Autodesk Inventor part; units mm, degrees
(part 2 of 5)
  spline S5 degree 5 poles (3.499, 4.4219) (3.499, 4.422) (3.4991, 4.4221) (3.4992, 4.4222) (3.4994, 4.4225) (3.4998, 4.423) (3.5001, 4.4234) (3.5005, 4.424) (3.501, 4.4246) (3.5015, 4.4253) (3.502, 4.426) (3.5026, 4.4268) (3.5032, 4.4277) (3.5039, 4.4286) (3.5046, 4.4296) (3.5053, 4.4307) (3.5061, 4.4318) (3.5069, 4.433) (3.5077, 4.4342) (3.5086, 4.4355) (3.5095, 4.4369) (3.5104, 4.4383) (3.5114, 4.4398) (3.5124, 4.4413) (3.5135, 4.4429) (3.5145, 4.4446) (3.5156, 4.4463) (3.5168, 4.4481) (3.5179, 4.4499) (3.5191, 4.4518) (3.5203, 4.4538) (3.5215, 4.4558) (3.5231, 4.4583) (3.5246, 4.4609) (3.5262, 4.4635) (3.5281, 4.4667) (3.53, 4.4701) (3.5317, 4.473) (3.5337, 4.4765) (3.5358, 4.4802) (3.5376, 4.4834) (3.5394, 4.4867) (3.5416, 4.4906) (3.5444, 4.4958) (3.5473, 4.5012) (3.5502, 4.5068) (3.5532, 4.5125) (3.5562, 4.5185) (3.5586, 4.5232) (3.561, 4.528) (3.5635, 4.533) (3.5663, 4.5387) (3.5687, 4.5439) (3.5709, 4.5484) (3.5734, 4.5538) (3.5759, 4.5592) (3.5781, 4.564) (3.5807, 4.5696) (3.5832, 4.5753) (3.5855, 4.5803) (3.5881, 4.5862) (3.5907, 4.5923) (3.5929, 4.5975) (3.5955, 4.6037) (3.5982, 4.61) (3.6004, 4.6155) (3.6031, 4.6219) (3.6057, 4.6285) (3.608, 4.6342) (3.6107, 4.641) (3.6133, 4.6478) (3.6156, 4.6537) (3.6183, 4.6607) (3.6209, 4.6679) (3.6232, 4.674) (3.6259, 4.6813) (3.6285, 4.6887) (3.6308, 4.6951) (3.6335, 4.7026) (3.6361, 4.7102) (3.6384, 4.7168) (3.641, 4.7246) (3.6437, 4.7325) (3.6459, 4.7393) (3.6485, 4.7474) (3.6511, 4.7555) (3.6533, 4.7626) (3.6559, 4.7708) (3.6585, 4.7792) (3.6607, 4.7865) (3.6632, 4.795) (3.6658, 4.8036) (3.6679, 4.8111) (3.6705, 4.8199) (3.6729, 4.8288) (3.6751, 4.8364) (3.6775, 4.8454) (3.68, 4.8545) (3.6821, 4.8624) (3.6845, 4.8717) (3.6869, 4.881) (3.6889, 4.8891) (3.6912, 4.8985) (3.6936, 4.9081) (3.6956, 4.9164) (3.6978, 4.9261) (3.7001, 4.9359) (3.702, 4.9443) (3.7043, 4.9543) (3.7065, 4.9643) (3.7083, 4.9729) (3.7105, 4.9831) (3.7126, 4.9933) (3.7144, 5.0021) (3.7165, 5.0125) (3.7185, 5.023) (3.7202, 5.032) (3.7222, 5.0425) (3.7242, 5.0532) (3.7258, 5.0624) (3.7277, 5.0732) (3.7296, 5.0841) (3.7312, 5.0934) (3.733, 5.1044) (3.7348, 5.1155) (3.7363, 5.1251) (3.738, 5.1363) (3.7397, 5.1475) (3.7411, 5.1572) (3.7427, 5.1686) (3.7443, 5.1801) (3.7456, 5.19) (3.7472, 5.2016) (3.7486, 5.2133) (3.7499, 5.2233) (3.7513, 5.2351) (3.7527, 5.247) (3.7538, 5.2572) (3.7551, 5.2692) (3.7564, 5.2812) (3.7574, 5.2916) (3.7586, 5.3037) (3.7598, 5.316) (3.7607, 5.3265) (3.7618, 5.3388) (3.7628, 5.3513) (3.7637, 5.3619) (3.7648, 5.3763) (3.7658, 5.3907) (3.7667, 5.4033) (3.7675, 5.4161) (3.7682, 5.4289) (3.7691, 5.4435) (3.7698, 5.4583) (3.7705, 5.4731) (3.7712, 5.4881) (3.7718, 5.505) (3.7722, 5.5163) (3.7726, 5.5276) (3.773, 5.5428) (3.7734, 5.5581) (3.7736, 5.5715) (3.7738, 5.585) (3.774, 5.5985) (3.7741, 5.6082) (3.7741, 5.6179) (3.7742, 5.6277) (3.7742, 5.6375) (3.7742, 5.6473) (3.7742, 5.6571) (3.7741, 5.667) (3.774, 5.6769) (3.7739, 5.6868) (3.7738, 5.6967) (3.7736, 5.7067) (3.7734, 5.7167) (3.7732, 5.7267) (3.7729, 5.7368) (3.7727, 5.7468) (3.7724, 5.757) (3.772, 5.7671) (3.7717, 5.7772) (3.7713, 5.7874) (3.7709, 5.7976) (3.7705, 5.8079) (3.77, 5.8181) (3.7695, 5.8284) (3.769, 5.8387) (3.7685, 5.849) (3.7677, 5.8635) (3.7669, 5.876) (3.7663, 5.8864) (3.7657, 5.8948) (3.7653, 5.901) knots 0 0 0 0 0 0 0.004167 0.008333 0.0125 0.016667 0.020833 0.025 0.029167 0.033333 0.0375 0.041667 0.045833 0.05 0.054167 0.058333 0.0625 0.066667 0.070833 0.075 0.079167 0.083333 0.0875 0.091667 0.095833 0.1 0.104167 0.108333 0.1125 0.116667 0.120833 0.125 0.129167 0.1375 0.141667 0.145833 0.154167 0.158333 0.1625 0.170833 0.175 0.179167 0.183333 0.191667 0.208333 0.2125 0.216667 0.220833 0.229167 0.2375 0.241667 0.245833 0.254167 0.258333 0.2625 0.270833 0.275 0.279167 0.2875 0.291667 0.295833 0.304167 0.308333 0.3125 0.320833 0.325 0.329167 0.3375 0.341667 0.345833 0.354167 0.358333 0.3625 0.370833 0.375 0.379167 0.3875 0.391667 0.395833 0.404167 0.408333 0.4125 0.420833 0.425 0.429167 0.4375 0.441667 0.445833 0.454167 0.458333 0.4625 0.470833 0.475 0.479167 0.4875 0.491667 0.495833 0.504167 0.508333 0.5125 0.520833 0.525 0.529167 0.5375 0.541667 0.545833 0.554167 0.558333 0.5625 0.570833 0.575 0.579167 0.5875 0.591667 0.595833 0.604167 0.608333 0.6125 0.620833 0.625 0.629167 0.6375 0.641667 0.645833 0.654167 0.658333 0.6625 0.670833 0.675 0.679167 0.6875 0.691667 0.695833 0.704167 0.708333 0.7125 0.720833 0.725 0.729167 0.7375 0.741667 0.745833 0.754167 0.758333 0.7625 0.770833 0.775 0.779167 0.791667 0.795833 0.8 0.804167 0.808333 0.825 0.829167 0.833333 0.8375 0.845833 0.85 0.854167 0.866667 0.870833 0.875 0.879167 0.883333 0.8875 0.891667 0.895833 0.9 0.904167 0.908333 0.9125 0.916667 0.920833 0.925 0.929167 0.933333 0.9375 0.941667 0.945833 0.95 0.954167 0.958333 0.9625 0.966667 0.970833 0.975 0.979167 0.983333 0.9875 1 1 1 1 1 1
  arc A5 (3.7653, 5.901) -> (3.2278, 6.2114) centre (0, 0) ccw
  spline S6 degree 5 poles (3.2278, 6.2114) (3.2221, 6.2086) (3.2146, 6.2049) (3.2053, 6.2003) (3.1941, 6.1947) (3.1812, 6.1881) (3.172, 6.1834) (3.1628, 6.1787) (3.1536, 6.174) (3.1445, 6.1692) (3.1354, 6.1645) (3.1264, 6.1598) (3.1174, 6.155) (3.1084, 6.1502) (3.0995, 6.1454) (3.0906, 6.1406) (3.0817, 6.1358) (3.0729, 6.131) (3.0641, 6.1262) (3.0554, 6.1214) (3.0466, 6.1165) (3.038, 6.1117) (3.0293, 6.1068) (3.0207, 6.1019) (3.0121, 6.0971) (3.0036, 6.0922) (2.9951, 6.0873) (2.9866, 6.0824) (2.9782, 6.0775) (2.9698, 6.0726) (2.9598, 6.0666) (2.9498, 6.0607) (2.9399, 6.0548) (2.9284, 6.0478) (2.917, 6.0409) (2.9072, 6.0349) (2.8975, 6.0289) (2.8879, 6.023) (2.8783, 6.017) (2.8688, 6.011) (2.8593, 6.0049) (2.8484, 5.9979) (2.8375, 5.9909) (2.8282, 5.9849) (2.8174, 5.9778) (2.8067, 5.9707) (2.7976, 5.9647) (2.7871, 5.9576) (2.7766, 5.9505) (2.7677, 5.9445) (2.7558, 5.9364) (2.7441, 5.9283) (2.734, 5.9212) (2.7239, 5.914) (2.711, 5.9049) (2.7011, 5.8978) (2.6912, 5.8907) (2.6815, 5.8836) (2.669, 5.8744) (2.6594, 5.8673) (2.6499, 5.8602) (2.6391, 5.852) (2.6285, 5.8439) (2.6205, 5.8378) (2.6113, 5.8307) (2.6022, 5.8236) (2.5945, 5.8175) (2.5855, 5.8104) (2.5766, 5.8033) (2.569, 5.7972) (2.5603, 5.7902) (2.5516, 5.7831) (2.5442, 5.777) (2.5357, 5.77) (2.5272, 5.7629) (2.5201, 5.7569) (2.5117, 5.7498) (2.5035, 5.7428) (2.4965, 5.7368) (2.4885, 5.7298) (2.4805, 5.7228) (2.4737, 5.7168) (2.4658, 5.7099) (2.458, 5.7029) (2.4514, 5.697) (2.4438, 5.69) (2.4362, 5.6831) (2.4298, 5.6772) (2.4224, 5.6704) (2.4151, 5.6635) (2.4089, 5.6577) (2.4017, 5.6508) (2.3946, 5.644) (2.3886, 5.6382) (2.3817, 5.6315) (2.3748, 5.6248) (2.369, 5.619) (2.3623, 5.6123) (2.3556, 5.6057) (2.35, 5.6) (2.3435, 5.5934) (2.3371, 5.5868) (2.3317, 5.5812) (2.3254, 5.5746) (2.3192, 5.5681) (2.314, 5.5626) (2.308, 5.5561) (2.302, 5.5497) (2.297, 5.5443) (2.2912, 5.5379) (2.2855, 5.5316) (2.2806, 5.5262) (2.2751, 5.52) (2.2696, 5.5138) (2.2649, 5.5085) (2.2596, 5.5023) (2.2543, 5.4962) (2.2499, 5.491) (2.2448, 5.485) (2.2398, 5.4791) (2.2355, 5.474) (2.2306, 5.4681) (2.2258, 5.4622) (2.2218, 5.4572) (2.2171, 5.4515) (2.2126, 5.4458) (2.2087, 5.4409) (2.2043, 5.4353) (2.1999, 5.4297) (2.1963, 5.425) (2.1921, 5.4195) (2.188, 5.4141) (2.1845, 5.4095) (2.1806, 5.4042) (2.1767, 5.399) (2.1734, 5.3945) (2.1697, 5.3894) (2.166, 5.3843) (2.1629, 5.38) (2.1594, 5.375) (2.156, 5.3701) (2.1531, 5.366) (2.1498, 5.3612) (2.1466, 5.3565) (2.1439, 5.3525) (2.1409, 5.348) (2.1379, 5.3435) (2.1354, 5.3397) (2.1326, 5.3353) (2.1298, 5.331) (2.1275, 5.3274) (2.1249, 5.3232) (2.1224, 5.3192) (2.1202, 5.3158) (2.1182, 5.3124) (2.1155, 5.308) (2.1133, 5.3043) (2.1108, 5.3001) (2.1084, 5.296) (2.1062, 5.2921) (2.1045, 5.2893) (2.1029, 5.2865) (2.1017, 5.2842) (2.1004, 5.2819) (2.0992, 5.2798) (2.0981, 5.2776) (2.0969, 5.2756) (2.0958, 5.2735) (2.0948, 5.2716) (2.0938, 5.2696) (2.0928, 5.2678) (2.0918, 5.266) (2.0909, 5.2642) (2.0901, 5.2625) (2.0892, 5.2609) (2.0884, 5.2593) (2.0877, 5.2577) (2.087, 5.2563) (2.0863, 5.2549) (2.0856, 5.2535) (2.085, 5.2522) (2.0844, 5.251) (2.0839, 5.2498) (2.0834, 5.2487) (2.0829, 5.2477) (2.0824, 5.2467) (2.082, 5.2458) (2.0817, 5.245) (2.0813, 5.2442) (2.081, 5.2435) (2.0807, 5.2429) (2.0805, 5.2422) (2.0803, 5.2418) (2.0801, 5.2415) (2.08, 5.2413) (2.08, 5.2411) knots -1 -1 -1 -1 -1 -1 -0.9875 -0.983333 -0.979167 -0.975 -0.970833 -0.966667 -0.9625 -0.958333 -0.954167 -0.95 -0.945833 -0.941667 -0.9375 -0.933333 -0.929167 -0.925 -0.920833 -0.916667 -0.9125 -0.908333 -0.904167 -0.9 -0.895833 -0.891667 -0.8875 -0.883333 -0.879167 -0.875 -0.870833 -0.8625 -0.858333 -0.854167 -0.845833 -0.841667 -0.8375 -0.833333 -0.829167 -0.820833 -0.816667 -0.8125 -0.804167 -0.8 -0.795833 -0.7875 -0.783333 -0.779167 -0.770833 -0.766667 -0.7625 -0.75 -0.745833 -0.741667 -0.7375 -0.725 -0.720833 -0.716667 -0.7125 -0.7 -0.695833 -0.691667 -0.683333 -0.679167 -0.675 -0.666667 -0.6625 -0.658333 -0.65 -0.645833 -0.641667 -0.633333 -0.629167 -0.625 -0.616667 -0.6125 -0.608333 -0.6 -0.595833 -0.591667 -0.583333 -0.579167 -0.575 -0.566667 -0.5625 -0.558333 -0.55 -0.545833 -0.541667 -0.533333 -0.529167 -0.525 -0.516667 -0.5125 -0.508333 -0.5 -0.495833 -0.491667 -0.483333 -0.479167 -0.475 -0.466667 -0.4625 -0.458333 -0.45 -0.445833 -0.441667 -0.433333 -0.429167 -0.425 -0.416667 -0.4125 -0.408333 -0.4 -0.395833 -0.391667 -0.383333 -0.379167 -0.375 -0.366667 -0.3625 -0.358333 -0.35 -0.345833 -0.341667 -0.333333 -0.329167 -0.325 -0.316667 -0.3125 -0.308333 -0.3 -0.295833 -0.291667 -0.283333 -0.279167 -0.275 -0.266667 -0.2625 -0.258333 -0.25 -0.245833 -0.241667 -0.233333 -0.229167 -0.225 -0.216667 -0.2125 -0.208333 -0.2 -0.195833 -0.191667 -0.183333 -0.179167 -0.175 -0.170833 -0.158333 -0.154167 -0.145833 -0.141667 -0.1375 -0.133333 -0.129167 -0.125 -0.120833 -0.116667 -0.1125 -0.108333 -0.104167 -0.1 -0.095833 -0.091667 -0.0875 -0.083333 -0.079167 -0.075 -0.070833 -0.066667 -0.0625 -0.058333 -0.054167 -0.05 -0.045833 -0.041667 -0.0375 -0.033333 -0.029167 -0.025 -0.020833 -0.016667 -0.0125 -0.008333 0 0 0 0 0 0
  line L6 (2.08, 5.2411) -> (1.7521, 4.415)
  arc A6 (1.7521, 4.415) -> (0.6901, 4.6996) centre (0, 0) ccw
  line L7 (0.6901, 4.6996) -> (0.8192, 5.579)
  spline S7 degree 5 poles (0.8192, 5.579) (0.8193, 5.579) (0.8193, 5.5792) (0.8193, 5.5794) (0.8193, 5.5797) (0.8194, 5.5803) (0.8195, 5.5809) (0.8196, 5.5815) (0.8196, 5.5823) (0.8197, 5.5831) (0.8198, 5.584) (0.8199, 5.585) (0.82, 5.5861) (0.8201, 5.5872) (0.8202, 5.5884) (0.8203, 5.5897) (0.8204, 5.5911) (0.8206, 5.5925) (0.8207, 5.594) (0.8208, 5.5955) (0.8209, 5.5972) (0.821, 5.5989) (0.8211, 5.6007) (0.8212, 5.6025) (0.8213, 5.6044) (0.8214, 5.6064) (0.8215, 5.6084) (0.8216, 5.6105) (0.8216, 5.6127) (0.8217, 5.6149) (0.8218, 5.6172) (0.8218, 5.6196) (0.8219, 5.6225) (0.822, 5.6255) (0.822, 5.6286) (0.822, 5.6323) (0.8221, 5.6362) (0.8221, 5.6396) (0.8221, 5.6437) (0.822, 5.6478) (0.822, 5.6515) (0.8219, 5.6559) (0.8218, 5.6604) (0.8217, 5.6644) (0.8215, 5.6691) (0.8214, 5.6739) (0.8212, 5.6781) (0.821, 5.6831) (0.8207, 5.6883) (0.8205, 5.6927) (0.8202, 5.6981) (0.8198, 5.7035) (0.8195, 5.7082) (0.8191, 5.7138) (0.8187, 5.7195) (0.8183, 5.7245) (0.8178, 5.7304) (0.8172, 5.7364) (0.8168, 5.7416) (0.8162, 5.7477) (0.8155, 5.754) (0.8149, 5.7594) (0.8142, 5.7658) (0.8135, 5.7723) (0.8128, 5.778) (0.812, 5.7847) (0.8111, 5.7915) (0.8103, 5.7973) (0.8094, 5.8042) (0.8084, 5.8113) (0.8075, 5.8173) (0.8064, 5.8245) (0.8053, 5.8318) (0.8043, 5.8381) (0.8031, 5.8455) (0.8019, 5.853) (0.8008, 5.8594) (0.7995, 5.8671) (0.7981, 5.8748) (0.7969, 5.8814) (0.7954, 5.8893) (0.7939, 5.8972) (0.7925, 5.9041) (0.7909, 5.9122) (0.7892, 5.9203) (0.7878, 5.9273) (0.786, 5.9356) (0.7842, 5.944) (0.7826, 5.9512) (0.7807, 5.9596) (0.7787, 5.9682) (0.777, 5.9756) (0.775, 5.9842) (0.7728, 5.993) (0.771, 6.0005) (0.7688, 6.0094) (0.7665, 6.0183) (0.7645, 6.026) (0.7621, 6.035) (0.7597, 6.0441) (0.7576, 6.052) (0.755, 6.0612) (0.7524, 6.0705) (0.7501, 6.0785) (0.7474, 6.0879) (0.7447, 6.0973) (0.7423, 6.1055) (0.7394, 6.115) (0.7365, 6.1246) (0.7339, 6.1329) (0.7309, 6.1426) (0.7277, 6.1524) (0.725, 6.1608) (0.7218, 6.1707) (0.7185, 6.1806) (0.7157, 6.1892) (0.7123, 6.1992) (0.7088, 6.2093) (0.7058, 6.2179) (0.7023, 6.2281) (0.6986, 6.2383) (0.6955, 6.2471) (0.6917, 6.2574) (0.6879, 6.2677) (0.6846, 6.2766) (0.6807, 6.2871) (0.6767, 6.2976) (0.6732, 6.3066) (0.6691, 6.3171) (0.6649, 6.3277) (0.6613, 6.3369) (0.657, 6.3475) (0.6526, 6.3583) (0.6488, 6.3675) (0.6443, 6.3783) (0.6398, 6.3891) (0.6358, 6.3985) (0.6312, 6.4094) (0.6264, 6.4203) (0.6223, 6.4298) (0.6175, 6.4408) (0.6125, 6.4518) (0.6082, 6.4614) (0.6032, 6.4725) (0.5981, 6.4837) (0.5936, 6.4933) (0.5884, 6.5045) (0.5831, 6.5157) (0.5785, 6.5254) (0.5738, 6.5351) (0.5667, 6.5497) (0.5604, 6.5627) (0.5539, 6.5758) (0.5473, 6.5889) (0.539, 6.6053) (0.5331, 6.6169) (0.5271, 6.6285) (0.521, 6.64) (0.5131, 6.655) (0.5069, 6.6666) (0.5006, 6.6783) (0.4934, 6.6917) (0.486, 6.7051) (0.4804, 6.7152) (0.4748, 6.7253) (0.4691, 6.7354) (0.4644, 6.7439) (0.4595, 6.7523) (0.4547, 6.7608) (0.4498, 6.7693) (0.4449, 6.7778) (0.44, 6.7863) (0.435, 6.7948) (0.43, 6.8033) (0.4249, 6.8118) (0.4198, 6.8204) (0.4147, 6.8289) (0.4095, 6.8375) (0.4043, 6.8461) (0.3991, 6.8547) (0.3938, 6.8632) (0.3885, 6.8718) (0.3831, 6.8805) (0.3778, 6.8891) (0.3723, 6.8977) (0.3669, 6.9063) (0.3614, 6.915) (0.3559, 6.9236) (0.3503, 6.9323) (0.3447, 6.941) (0.3391, 6.9496) (0.3311, 6.9618) (0.3243, 6.9722) (0.3185, 6.9809) (0.3138, 6.9879) (0.3103, 6.9931) knots 0 0 0 0 0 0 0.004167 0.008333 0.0125 0.016667 0.020833 0.025 0.029167 0.033333 0.0375 0.041667 0.045833 0.05 0.054167 0.058333 0.0625 0.066667 0.070833 0.075 0.079167 0.083333 0.0875 0.091667 0.095833 0.1 0.104167 0.108333 0.1125 0.116667 0.120833 0.125 0.129167 0.1375 0.141667 0.145833 0.154167 0.158333 0.1625 0.170833 0.175 0.179167 0.1875 0.191667 0.195833 0.204167 0.208333 0.2125 0.220833 0.225 0.229167 0.2375 0.241667 0.245833 0.254167 0.258333 0.2625 0.270833 0.275 0.279167 0.2875 0.291667 0.295833 0.304167 0.308333 0.3125 0.320833 0.325 0.329167 0.3375 0.341667 0.345833 0.354167 0.358333 0.3625 0.370833 0.375 0.379167 0.3875 0.391667 0.395833 0.404167 0.408333 0.4125 0.420833 0.425 0.429167 0.4375 0.441667 0.445833 0.454167 0.458333 0.4625 0.470833 0.475 0.479167 0.4875 0.491667 0.495833 0.504167 0.508333 0.5125 0.520833 0.525 0.529167 0.5375 0.541667 0.545833 0.554167 0.558333 0.5625 0.570833 0.575 0.579167 0.5875 0.591667 0.595833 0.604167 0.608333 0.6125 0.620833 0.625 0.629167 0.6375 0.641667 0.645833 0.654167 0.658333 0.6625 0.670833 0.675 0.679167 0.6875 0.691667 0.695833 0.704167 0.708333 0.7125 0.720833 0.725 0.729167 0.7375 0.741667 0.745833 0.754167 0.758333 0.7625 0.770833 0.775 0.779167 0.783333 0.8 0.804167 0.808333 0.8125 0.825 0.829167 0.833333 0.8375 0.85 0.854167 0.858333 0.866667 0.870833 0.875 0.879167 0.883333 0.8875 0.891667 0.895833 0.9 0.904167 0.908333 0.9125 0.916667 0.920833 0.925 0.929167 0.933333 0.9375 0.941667 0.945833 0.95 0.954167 0.958333 0.9625 0.966667 0.970833 0.975 0.979167 0.983333 0.9875 1 1 1 1 1 1
  arc A7 (0.3103, 6.9931) -> (-0.3103, 6.9931) centre (0, 0) ccw
  spline S8 degree 5 poles (-0.3103, 6.9931) (-0.3138, 6.9879) (-0.3185, 6.9809) (-0.3243, 6.9722) (-0.3311, 6.9618) (-0.3391, 6.9496) (-0.3447, 6.941) (-0.3503, 6.9323) (-0.3559, 6.9236) (-0.3614, 6.915) (-0.3669, 6.9063) (-0.3723, 6.8977) (-0.3778, 6.8891) (-0.3831, 6.8805) (-0.3885, 6.8718) (-0.3938, 6.8632) (-0.3991, 6.8547) (-0.4043, 6.8461) (-0.4095, 6.8375) (-0.4147, 6.8289) (-0.4198, 6.8204) (-0.4249, 6.8118) (-0.43, 6.8033) (-0.435, 6.7948) (-0.44, 6.7863) (-0.4449, 6.7778) (-0.4498, 6.7693) (-0.4547, 6.7608) (-0.4595, 6.7523) (-0.4644, 6.7439) (-0.4701, 6.7337) (-0.4758, 6.7236) (-0.4814, 6.7135) (-0.4879, 6.7018) (-0.4943, 6.69) (-0.4997, 6.68) (-0.5051, 6.67) (-0.5105, 6.66) (-0.5158, 6.65) (-0.521, 6.64) (-0.5262, 6.6301) (-0.5322, 6.6185) (-0.5381, 6.607) (-0.5432, 6.5971) (-0.549, 6.5856) (-0.5547, 6.5742) (-0.5595, 6.5644) (-0.5651, 6.553) (-0.5707, 6.5416) (-0.5754, 6.5319) (-0.5808, 6.5206) (-0.5861, 6.5093) (-0.5906, 6.4997) (-0.5966, 6.4868) (-0.6025, 6.4741) (-0.6075, 6.4629) (-0.6125, 6.4518) (-0.6189, 6.4376) (-0.6237, 6.4266) (-0.6285, 6.4156) (-0.6332, 6.4047) (-0.6391, 6.3907) (-0.6437, 6.3798) (-0.6482, 6.369) (-0.6533, 6.3567) (-0.6582, 6.3445) (-0.6619, 6.3353) (-0.6661, 6.3247) (-0.6703, 6.3141) (-0.6738, 6.3051) (-0.6778, 6.2946) (-0.6818, 6.2841) (-0.6851, 6.2752) (-0.689, 6.2648) (-0.6928, 6.2544) (-0.696, 6.2456) (-0.6997, 6.2354) (-0.7033, 6.2252) (-0.7063, 6.2165) (-0.7098, 6.2064) (-0.7133, 6.1963) (-0.7162, 6.1877) (-0.7195, 6.1778) (-0.7227, 6.1679) (-0.7255, 6.1594) (-0.7286, 6.1496) (-0.7317, 6.1399) (-0.7343, 6.1315) (-0.7373, 6.1219) (-0.7402, 6.1123) (-0.7427, 6.1041) (-0.7455, 6.0946) (-0.7482, 6.0852) (-0.7505, 6.0772) (-0.7532, 6.0678) (-0.7557, 6.0586) (-0.7579, 6.0507) (-0.7604, 6.0415) (-0.7628, 6.0325) (-0.7648, 6.0247) (-0.7671, 6.0157) (-0.7694, 6.0068) (-0.7713, 5.9993) (-0.7734, 5.9905) (-0.7755, 5.9818) (-0.7773, 5.9743) (-0.7793, 5.9657) (-0.7813, 5.9572) (-0.7829, 5.95) (-0.7847, 5.9416) (-0.7865, 5.9332) (-0.788, 5.9262) (-0.7897, 5.918) (-0.7914, 5.9098) (-0.7927, 5.9029) (-0.7943, 5.895) (-0.7958, 5.887) (-0.7971, 5.8803) (-0.7985, 5.8726) (-0.7998, 5.8649) (-0.801, 5.8583) (-0.8023, 5.8508) (-0.8035, 5.8433) (-0.8045, 5.837) (-0.8057, 5.8297) (-0.8068, 5.8225) (-0.8077, 5.8163) (-0.8087, 5.8093) (-0.8097, 5.8023) (-0.8105, 5.7963) (-0.8114, 5.7895) (-0.8122, 5.7828) (-0.8129, 5.7771) (-0.8137, 5.7705) (-0.8144, 5.764) (-0.815, 5.7585) (-0.8157, 5.7522) (-0.8163, 5.7459) (-0.8168, 5.7407) (-0.8174, 5.7346) (-0.8179, 5.7287) (-0.8183, 5.7236) (-0.8188, 5.7179) (-0.8192, 5.7122) (-0.8196, 5.7074) (-0.8199, 5.7019) (-0.8202, 5.6965) (-0.8205, 5.692) (-0.8208, 5.6868) (-0.821, 5.6817) (-0.8212, 5.6774) (-0.8214, 5.6725) (-0.8216, 5.6677) (-0.8217, 5.6637) (-0.8218, 5.6598) (-0.8219, 5.6546) (-0.822, 5.6503) (-0.822, 5.6454) (-0.8221, 5.6407) (-0.8221, 5.6362) (-0.8221, 5.6329) (-0.822, 5.6297) (-0.822, 5.6271) (-0.822, 5.6245) (-0.8219, 5.622) (-0.8218, 5.6196) (-0.8218, 5.6172) (-0.8217, 5.6149) (-0.8216, 5.6127) (-0.8216, 5.6105) (-0.8215, 5.6084) (-0.8214, 5.6064) (-0.8213, 5.6044) (-0.8212, 5.6025) (-0.8211, 5.6007) (-0.821, 5.5989) (-0.8209, 5.5972) (-0.8208, 5.5955) (-0.8207, 5.594) (-0.8206, 5.5925) (-0.8204, 5.5911) (-0.8203, 5.5897) (-0.8202, 5.5884) (-0.8201, 5.5872) (-0.82, 5.5861) (-0.8199, 5.585) (-0.8198, 5.584) (-0.8197, 5.5831) (-0.8196, 5.5823) (-0.8196, 5.5815) (-0.8195, 5.5809) (-0.8194, 5.5801) (-0.8193, 5.5796) (-0.8193, 5.5793) (-0.8193, 5.5791) (-0.8192, 5.579) knots -1 -1 -1 -1 -1 -1 -0.9875 -0.983333 -0.979167 -0.975 -0.970833 -0.966667 -0.9625 -0.958333 -0.954167 -0.95 -0.945833 -0.941667 -0.9375 -0.933333 -0.929167 -0.925 -0.920833 -0.916667 -0.9125 -0.908333 -0.904167 -0.9 -0.895833 -0.891667 -0.8875 -0.883333 -0.879167 -0.875 -0.870833 -0.8625 -0.858333 -0.854167 -0.845833 -0.841667 -0.8375 -0.833333 -0.829167 -0.820833 -0.816667 -0.8125 -0.804167 -0.8 -0.795833 -0.7875 -0.783333 -0.779167 -0.770833 -0.766667 -0.7625 -0.754167 -0.75 -0.745833 -0.733333 -0.729167 -0.725 -0.720833 -0.708333 -0.704167 -0.7 -0.695833 -0.683333 -0.679167 -0.675 -0.666667 -0.6625 -0.658333 -0.65 -0.645833 -0.641667 -0.633333 -0.629167 -0.625 -0.616667 -0.6125 -0.608333 -0.6 -0.595833 -0.591667 -0.583333 -0.579167 -0.575 -0.566667 -0.5625 -0.558333 -0.55 -0.545833 -0.541667 -0.533333 -0.529167 -0.525 -0.516667 -0.5125 -0.508333 -0.5 -0.495833 -0.491667 -0.483333 -0.479167 -0.475 -0.466667 -0.4625 -0.458333 -0.45 -0.445833 -0.441667 -0.433333 -0.429167 -0.425 -0.416667 -0.4125 -0.408333 -0.4 -0.395833 -0.391667 -0.383333 -0.379167 -0.375 -0.366667 -0.3625 -0.358333 -0.35 -0.345833 -0.341667 -0.333333 -0.329167 -0.325 -0.316667 -0.3125 -0.308333 -0.3 -0.295833 -0.291667 -0.283333 -0.279167 -0.275 -0.266667 -0.2625 -0.258333 -0.25 -0.245833 -0.241667 -0.233333 -0.229167 -0.225 -0.216667 -0.2125 -0.208333 -0.2 -0.195833 -0.191667 -0.183333 -0.179167 -0.175 -0.170833 -0.158333 -0.154167 -0.145833 -0.141667 -0.1375 -0.133333 -0.129167 -0.125 -0.120833 -0.116667 -0.1125 -0.108333 -0.104167 -0.1 -0.095833 -0.091667 -0.0875 -0.083333 -0.079167 -0.075 -0.070833 -0.066667 -0.0625 -0.058333 -0.054167 -0.05 -0.045833 -0.041667 -0.0375 -0.033333 -0.029167 -0.025 -0.020833 -0.016667 -0.0125 -0.008333 0 0 0 0 0 0
  line L8 (-0.8192, 5.579) -> (-0.6901, 4.6996)
  arc A8 (-0.6901, 4.6996) -> (-1.7521, 4.415) centre (0, 0) ccw construction
  line L9 (-1.7521, 4.415) -> (-2.08, 5.2411) construction
  spline S9 degree 5 poles (-2.08, 5.2411) (-2.08, 5.2412) (-2.0801, 5.2413) (-2.0802, 5.2415) (-2.0803, 5.2419) (-2.0805, 5.2424) (-2.0807, 5.2429) (-2.081, 5.2435) (-2.0813, 5.2442) (-2.0817, 5.245) (-2.082, 5.2458) (-2.0824, 5.2467) (-2.0829, 5.2477) (-2.0834, 5.2487) (-2.0839, 5.2498) (-2.0844, 5.251) (-2.085, 5.2522) (-2.0856, 5.2535) (-2.0863, 5.2549) (-2.087, 5.2563) (-2.0877, 5.2577) (-2.0884, 5.2593) (-2.0892, 5.2609) (-2.0901, 5.2625) (-2.0909, 5.2642) (-2.0918, 5.266) (-2.0928, 5.2678) (-2.0938, 5.2696) (-2.0948, 5.2716) (-2.0958, 5.2735) (-2.0969, 5.2756) (-2.0981, 5.2776) (-2.0995, 5.2802) (-2.1009, 5.2828) (-2.1024, 5.2855) (-2.1043, 5.2888) (-2.1062, 5.2921) (-2.1079, 5.2951) (-2.1099, 5.2986) (-2.112, 5.3022) (-2.1139, 5.3053) (-2.1162, 5.3091) (-2.1185, 5.313) (-2.1206, 5.3163) (-2.1231, 5.3203) (-2.1256, 5.3244) (-2.1279, 5.328) (-2.1306, 5.3322) (-2.1334, 5.3365) (-2.1358, 5.3403) (-2.1387, 5.3447) (-2.1418, 5.3493) (-2.1444, 5.3532) (-2.1475, 5.3579) (-2.1508, 5.3626) (-2.1536, 5.3667) (-2.157, 5.3715) (-2.1604, 5.3764) (-2.1635, 5.3807) (-2.167, 5.3857) (-2.1707, 5.3908) (-2.1739, 5.3953) (-2.1778, 5.4005) (-2.1817, 5.4057) (-2.1851, 5.4103) (-2.1891, 5.4157) (-2.1933, 5.4211) (-2.1969, 5.4258) (-2.2012, 5.4313) (-2.2055, 5.4369) (-2.2093, 5.4417) (-2.2139, 5.4474) (-2.2184, 5.4531) (-2.2224, 5.4581) (-2.2272, 5.4639) (-2.232, 5.4698) (-2.2362, 5.4748) (-2.2412, 5.4808) (-2.2462, 5.4867) (-2.2506, 5.4919) (-2.2558, 5.498) (-2.2611, 5.5041) (-2.2657, 5.5093) (-2.2711, 5.5155) (-2.2766, 5.5217) (-2.2814, 5.5271) (-2.2871, 5.5334) (-2.2928, 5.5397) (-2.2978, 5.5452) (-2.3037, 5.5516) (-2.3097, 5.558) (-2.3149, 5.5635) (-2.321, 5.57) (-2.3272, 5.5765) (-2.3326, 5.5821) (-2.3389, 5.5887) (-2.3454, 5.5952) (-2.3509, 5.6009) (-2.3575, 5.6076) (-2.3642, 5.6142) (-2.3699, 5.62) (-2.3767, 5.6267) (-2.3836, 5.6334) (-2.3896, 5.6392) (-2.3966, 5.646) (-2.4038, 5.6528) (-2.4099, 5.6586) (-2.4172, 5.6655) (-2.4245, 5.6723) (-2.4309, 5.6782) (-2.4384, 5.6851) (-2.446, 5.692) (-2.4525, 5.698) (-2.4602, 5.7049) (-2.468, 5.7118) (-2.4748, 5.7178) (-2.4827, 5.7248) (-2.4908, 5.7318) (-2.4977, 5.7378) (-2.5059, 5.7448) (-2.5141, 5.7518) (-2.5212, 5.7579) (-2.5296, 5.7649) (-2.5381, 5.772) (-2.5454, 5.778) (-2.5541, 5.7851) (-2.5628, 5.7922) (-2.5703, 5.7982) (-2.5791, 5.8053) (-2.588, 5.8124) (-2.5957, 5.8185) (-2.6048, 5.8256) (-2.614, 5.8327) (-2.6218, 5.8388) (-2.6311, 5.8459) (-2.6405, 5.8531) (-2.6486, 5.8592) (-2.6581, 5.8663) (-2.6677, 5.8734) (-2.6759, 5.8795) (-2.6857, 5.8866) (-2.6955, 5.8937) (-2.7039, 5.8998) (-2.7139, 5.9069) (-2.7239, 5.914) (-2.7325, 5.9201) (-2.7427, 5.9272) (-2.7529, 5.9343) (-2.7617, 5.9404) (-2.7706, 5.9465) (-2.784, 5.9556) (-2.7961, 5.9637) (-2.8082, 5.9718) (-2.8205, 5.9798) (-2.8359, 5.9899) (-2.8468, 5.9969) (-2.8578, 6.0039) (-2.8688, 6.011) (-2.8847, 6.021) (-2.8975, 6.0289) (-2.9104, 6.0369) (-2.9235, 6.0449) (-2.9366, 6.0528) (-2.9448, 6.0577) (-2.9531, 6.0627) (-2.9614, 6.0676) (-2.9698, 6.0726) (-2.9782, 6.0775) (-2.9866, 6.0824) (-2.9951, 6.0873) (-3.0036, 6.0922) (-3.0121, 6.0971) (-3.0207, 6.1019) (-3.0293, 6.1068) (-3.038, 6.1117) (-3.0466, 6.1165) (-3.0554, 6.1214) (-3.0641, 6.1262) (-3.0729, 6.131) (-3.0817, 6.1358) (-3.0906, 6.1406) (-3.0995, 6.1454) (-3.1084, 6.1502) (-3.1174, 6.155) (-3.1264, 6.1598) (-3.1354, 6.1645) (-3.1445, 6.1692) (-3.1536, 6.174) (-3.1628, 6.1787) (-3.172, 6.1834) (-3.1812, 6.1881) (-3.1941, 6.1947) (-3.2053, 6.2003) (-3.2146, 6.2049) (-3.2221, 6.2086) (-3.2278, 6.2114) knots 0 0 0 0 0 0 0.004167 0.008333 0.0125 0.016667 0.020833 0.025 0.029167 0.033333 0.0375 0.041667 0.045833 0.05 0.054167 0.058333 0.0625 0.066667 0.070833 0.075 0.079167 0.083333 0.0875 0.091667 0.095833 0.1 0.104167 0.108333 0.1125 0.116667 0.120833 0.125 0.129167 0.1375 0.141667 0.145833 0.154167 0.158333 0.1625 0.170833 0.175 0.179167 0.1875 0.191667 0.195833 0.204167 0.208333 0.2125 0.220833 0.225 0.229167 0.2375 0.241667 0.245833 0.254167 0.258333 0.2625 0.270833 0.275 0.279167 0.2875 0.291667 0.295833 0.304167 0.308333 0.3125 0.320833 0.325 0.329167 0.3375 0.341667 0.345833 0.354167 0.358333 0.3625 0.370833 0.375 0.379167 0.3875 0.391667 0.395833 0.404167 0.408333 0.4125 0.420833 0.425 0.429167 0.4375 0.441667 0.445833 0.454167 0.458333 0.4625 0.470833 0.475 0.479167 0.4875 0.491667 0.495833 0.504167 0.508333 0.5125 0.520833 0.525 0.529167 0.5375 0.541667 0.545833 0.554167 0.558333 0.5625 0.570833 0.575 0.579167 0.5875 0.591667 0.595833 0.604167 0.608333 0.6125 0.620833 0.625 0.629167 0.6375 0.641667 0.645833 0.654167 0.658333 0.6625 0.670833 0.675 0.679167 0.6875 0.691667 0.695833 0.704167 0.708333 0.7125 0.720833 0.725 0.729167 0.7375 0.741667 0.745833 0.754167 0.758333 0.7625 0.770833 0.775 0.779167 0.783333 0.8 0.804167 0.808333 0.8125 0.825 0.829167 0.833333 0.8375 0.854167 0.858333 0.8625 0.866667 0.870833 0.875 0.879167 0.883333 0.8875 0.891667 0.895833 0.9 0.904167 0.908333 0.9125 0.916667 0.920833 0.925 0.929167 0.933333 0.9375 0.941667 0.945833 0.95 0.954167 0.958333 0.9625 0.966667 0.970833 0.975 0.979167 0.983333 0.9875 1 1 1 1 1 1 construction
  arc A9 (-3.2278, 6.2114) -> (-3.7653, 5.901) centre (0, 0) ccw construction
  spline S10 degree 5 poles (-3.7653, 5.901) (-3.7657, 5.8948) (-3.7663, 5.8864) (-3.7669, 5.876) (-3.7677, 5.8635) (-3.7685, 5.849) (-3.769, 5.8387) (-3.7695, 5.8284) (-3.77, 5.8181) (-3.7705, 5.8079) (-3.7709, 5.7976) (-3.7713, 5.7874) (-3.7717, 5.7772) (-3.772, 5.7671) (-3.7724, 5.757) (-3.7727, 5.7468) (-3.7729, 5.7368) (-3.7732, 5.7267) (-3.7734, 5.7167) (-3.7736, 5.7067) (-3.7738, 5.6967) (-3.7739, 5.6868) (-3.774, 5.6769) (-3.7741, 5.667) (-3.7742, 5.6571) (-3.7742, 5.6473) (-3.7742, 5.6375) (-3.7742, 5.6277) (-3.7741, 5.6179) (-3.7741, 5.6082) (-3.774, 5.5966) (-3.7738, 5.585) (-3.7736, 5.5734) (-3.7734, 5.56) (-3.7731, 5.5466) (-3.7728, 5.5352) (-3.7724, 5.5238) (-3.7721, 5.5125) (-3.7717, 5.5012) (-3.7712, 5.4899) (-3.7708, 5.4787) (-3.7702, 5.4657) (-3.7695, 5.4528) (-3.769, 5.4417) (-3.7682, 5.4288) (-3.7675, 5.4161) (-3.7668, 5.4051) (-3.7659, 5.3925) (-3.765, 5.3799) (-3.7642, 5.3691) (-3.7631, 5.3548) (-3.762, 5.3406) (-3.7609, 5.3283) (-3.7598, 5.316) (-3.7583, 5.3003) (-3.7571, 5.2881) (-3.7559, 5.276) (-3.7546, 5.264) (-3.7529, 5.2487) (-3.7515, 5.2368) (-3.7501, 5.225) (-3.7486, 5.2133) (-3.7467, 5.1983) (-3.7452, 5.1867) (-3.7436, 5.1752) (-3.7418, 5.1621) (-3.7399, 5.1491) (-3.7385, 5.1395) (-3.7368, 5.1282) (-3.735, 5.1171) (-3.7335, 5.1076) (-3.7317, 5.0966) (-3.7299, 5.0856) (-3.7283, 5.0763) (-3.7264, 5.0655) (-3.7245, 5.0547) (-3.7228, 5.0456) (-3.7208, 5.035) (-3.7188, 5.0245) (-3.717, 5.0155) (-3.715, 5.0051) (-3.7129, 4.9948) (-3.7111, 4.986) (-3.7089, 4.9758) (-3.7068, 4.9657) (-3.7049, 4.9571) (-3.7027, 4.9472) (-3.7004, 4.9373) (-3.6985, 4.9289) (-3.6962, 4.9191) (-3.6939, 4.9095) (-3.6919, 4.9013) (-3.6896, 4.8918) (-3.6872, 4.8823) (-3.6852, 4.8743) (-3.6828, 4.865) (-3.6803, 4.8559) (-3.6782, 4.848) (-3.6758, 4.839) (-3.6733, 4.83) (-3.6712, 4.8224) (-3.6687, 4.8136) (-3.6661, 4.8049) (-3.664, 4.7975) (-3.6614, 4.7889) (-3.6589, 4.7804) (-3.6567, 4.7732) (-3.6541, 4.7649) (-3.6515, 4.7567) (-3.6493, 4.7497) (-3.6466, 4.7416) (-3.644, 4.7336) (-3.6418, 4.7269) (-3.6391, 4.719) (-3.6365, 4.7113) (-3.6342, 4.7048) (-3.6316, 4.6972) (-3.6289, 4.6897) (-3.6266, 4.6834) (-3.624, 4.6761) (-3.6213, 4.6689) (-3.619, 4.6628) (-3.6164, 4.6557) (-3.6137, 4.6488) (-3.6114, 4.6429) (-3.6088, 4.6361) (-3.6061, 4.6295) (-3.6038, 4.6238) (-3.6012, 4.6173) (-3.5985, 4.6109) (-3.5963, 4.6055) (-3.5937, 4.5993) (-3.591, 4.5931) (-3.5888, 4.588) (-3.5862, 4.582) (-3.5836, 4.5762) (-3.5814, 4.5712) (-3.5788, 4.5656) (-3.5763, 4.56) (-3.5741, 4.5553) (-3.5716, 4.5499) (-3.5691, 4.5447) (-3.567, 4.5402) (-3.5645, 4.5351) (-3.5621, 4.5301) (-3.56, 4.526) (-3.5576, 4.5212) (-3.5552, 4.5165) (-3.5532, 4.5126) (-3.5509, 4.5081) (-3.5486, 4.5037) (-3.5467, 4.5) (-3.5444, 4.4958) (-3.5422, 4.4917) (-3.5403, 4.4883) (-3.5382, 4.4845) (-3.5361, 4.4807) (-3.5343, 4.4776) (-3.5323, 4.474) (-3.5303, 4.4705) (-3.5286, 4.4677) (-3.527, 4.4649) (-3.5254, 4.4622) (-3.5241, 4.46) (-3.5228, 4.4579) (-3.5215, 4.4558) (-3.5203, 4.4538) (-3.5191, 4.4518) (-3.5179, 4.4499) (-3.5168, 4.4481) (-3.5156, 4.4463) (-3.5145, 4.4446) (-3.5135, 4.4429) (-3.5124, 4.4413) (-3.5114, 4.4398) (-3.5104, 4.4383) (-3.5095, 4.4369) (-3.5086, 4.4355) (-3.5077, 4.4342) (-3.5069, 4.433) (-3.5061, 4.4318) (-3.5053, 4.4307) (-3.5046, 4.4296) (-3.5039, 4.4286) (-3.5032, 4.4277) (-3.5026, 4.4268) (-3.502, 4.426) (-3.5015, 4.4253) (-3.501, 4.4246) (-3.5005, 4.424) (-3.5001, 4.4234) (-3.4997, 4.4229) (-3.4994, 4.4224) (-3.4992, 4.4222) (-3.499, 4.422) (-3.499, 4.4219) knots -1 -1 -1 -1 -1 -1 -0.9875 -0.983333 -0.979167 -0.975 -0.970833 -0.966667 -0.9625 -0.958333 -0.954167 -0.95 -0.945833 -0.941667 -0.9375 -0.933333 -0.929167 -0.925 -0.920833 -0.916667 -0.9125 -0.908333 -0.904167 -0.9 -0.895833 -0.891667 -0.8875 -0.883333 -0.879167 -0.875 -0.870833 -0.8625 -0.858333 -0.854167 -0.845833 -0.841667 -0.8375 -0.833333 -0.829167 -0.820833 -0.816667 -0.8125 -0.804167 -0.8 -0.795833 -0.7875 -0.783333 -0.779167 -0.770833 -0.766667 -0.7625 -0.75 -0.745833 -0.741667 -0.7375 -0.725 -0.720833 -0.716667 -0.7125 -0.7 -0.695833 -0.691667 -0.6875 -0.675 -0.670833 -0.666667 -0.658333 -0.654167 -0.65 -0.641667 -0.6375 -0.633333 -0.625 -0.620833 -0.616667 -0.608333 -0.604167 -0.6 -0.591667 -0.5875 -0.583333 -0.575 -0.570833 -0.566667 -0.558333 -0.554167 -0.55 -0.541667 -0.5375 -0.533333 -0.525 -0.520833 -0.516667 -0.508333 -0.504167 -0.5 -0.491667 -0.4875 -0.483333 -0.475 -0.470833 -0.466667 -0.458333 -0.454167 -0.45 -0.441667 -0.4375 -0.433333 -0.425 -0.420833 -0.416667 -0.408333 -0.404167 -0.4 -0.391667 -0.3875 -0.383333 -0.375 -0.370833 -0.366667 -0.358333 -0.354167 -0.35 -0.341667 -0.3375 -0.333333 -0.325 -0.320833 -0.316667 -0.308333 -0.304167 -0.3 -0.291667 -0.2875 -0.283333 -0.275 -0.270833 -0.266667 -0.258333 -0.254167 -0.25 -0.241667 -0.2375 -0.233333 -0.225 -0.220833 -0.216667 -0.208333 -0.204167 -0.2 -0.191667 -0.1875 -0.183333 -0.175 -0.170833 -0.166667 -0.158333 -0.154167 -0.15 -0.141667 -0.1375 -0.133333 -0.129167 -0.125 -0.120833 -0.116667 -0.1125 -0.108333 -0.104167 -0.1 -0.095833 -0.091667 -0.0875 -0.083333 -0.079167 -0.075 -0.070833 -0.066667 -0.0625 -0.058333 -0.054167 -0.05 -0.045833 -0.041667 -0.0375 -0.033333 -0.029167 -0.025 -0.020833 -0.016667 -0.0125 -0.008333 0 0 0 0 0 0 construction
  line L10 (-3.499, 4.4219) -> (-2.9475, 3.7249) construction
  arc A10 (-2.9475, 3.7249) -> (-3.7249, 2.9475) centre (0, 0) ccw
  line L11 (-3.7249, 2.9475) -> (-4.4219, 3.499)
  spline S11 degree 5 poles (-4.4219, 3.499) (-4.422, 3.499) (-4.4221, 3.4991) (-4.4222, 3.4992) (-4.4225, 3.4994) (-4.423, 3.4998) (-4.4234, 3.5001) (-4.424, 3.5005) (-4.4246, 3.501) (-4.4253, 3.5015) (-4.426, 3.502) (-4.4268, 3.5026) (-4.4277, 3.5032) (-4.4286, 3.5039) (-4.4296, 3.5046) (-4.4307, 3.5053) (-4.4318, 3.5061) (-4.433, 3.5069) (-4.4342, 3.5077) (-4.4355, 3.5086) (-4.4369, 3.5095) (-4.4383, 3.5104) (-4.4398, 3.5114) (-4.4413, 3.5124) (-4.4429, 3.5135) (-4.4446, 3.5145) (-4.4463, 3.5156) (-4.4481, 3.5168) (-4.4499, 3.5179) (-4.4518, 3.5191) (-4.4538, 3.5203) (-4.4558, 3.5215) (-4.4583, 3.5231) (-4.4609, 3.5246) (-4.4635, 3.5262) (-4.4667, 3.5281) (-4.4701, 3.53) (-4.473, 3.5317) (-4.4765, 3.5337) (-4.4802, 3.5358) (-4.4834, 3.5376) (-4.4867, 3.5394) (-4.4906, 3.5416) (-4.4958, 3.5444) (-4.5012, 3.5473) (-4.5068, 3.5502) (-4.5125, 3.5532) (-4.5185, 3.5562) (-4.5232, 3.5586) (-4.528, 3.561) (-4.533, 3.5635) (-4.5387, 3.5663) (-4.5439, 3.5687) (-4.5484, 3.5709) (-4.5538, 3.5734) (-4.5592, 3.5759) (-4.564, 3.5781) (-4.5696, 3.5807) (-4.5753, 3.5832) (-4.5803, 3.5855) (-4.5862, 3.5881) (-4.5923, 3.5907) (-4.5975, 3.5929) (-4.6037, 3.5955) (-4.61, 3.5982) (-4.6155, 3.6004) (-4.6219, 3.6031) (-4.6285, 3.6057) (-4.6342, 3.608) (-4.641, 3.6107) (-4.6478, 3.6133) (-4.6537, 3.6156) (-4.6607, 3.6183) (-4.6679, 3.6209) (-4.674, 3.6232) (-4.6813, 3.6259) (-4.6887, 3.6285) (-4.6951, 3.6308) (-4.7026, 3.6335) (-4.7102, 3.6361) (-4.7168, 3.6384) (-4.7246, 3.641) (-4.7325, 3.6437) (-4.7393, 3.6459) (-4.7474, 3.6485) (-4.7555, 3.6511) (-4.7626, 3.6533) (-4.7708, 3.6559) (-4.7792, 3.6585) (-4.7865, 3.6607) (-4.795, 3.6632) (-4.8036, 3.6658) (-4.8111, 3.6679) (-4.8199, 3.6705) (-4.8288, 3.6729) (-4.8364, 3.6751) (-4.8454, 3.6775) (-4.8545, 3.68) (-4.8624, 3.6821) (-4.8717, 3.6845) (-4.881, 3.6869) (-4.8891, 3.6889) (-4.8985, 3.6912) (-4.9081, 3.6936) (-4.9164, 3.6956) (-4.9261, 3.6978) (-4.9359, 3.7001) (-4.9443, 3.702) (-4.9543, 3.7043) (-4.9643, 3.7065) (-4.9729, 3.7083) (-4.9831, 3.7105) (-4.9933, 3.7126) (-5.0021, 3.7144) (-5.0125, 3.7165) (-5.023, 3.7185) (-5.032, 3.7202) (-5.0425, 3.7222) (-5.0532, 3.7242) (-5.0624, 3.7258) (-5.0732, 3.7277) (-5.0841, 3.7296) (-5.0934, 3.7312) (-5.1044, 3.733) (-5.1155, 3.7348) (-5.1251, 3.7363) (-5.1363, 3.738) (-5.1475, 3.7397) (-5.1572, 3.7411) (-5.1686, 3.7427) (-5.1801, 3.7443) (-5.19, 3.7456) (-5.2016, 3.7472) (-5.2133, 3.7486) (-5.2233, 3.7499) (-5.2351, 3.7513) (-5.247, 3.7527) (-5.2572, 3.7538) (-5.2692, 3.7551) (-5.2812, 3.7564) (-5.2916, 3.7574) (-5.3037, 3.7586) (-5.316, 3.7598) (-5.3265, 3.7607) (-5.3388, 3.7618) (-5.3513, 3.7628) (-5.3619, 3.7637) (-5.3763, 3.7648) (-5.3907, 3.7658) (-5.4033, 3.7667) (-5.4161, 3.7675) (-5.4289, 3.7682) (-5.4435, 3.7691) (-5.4583, 3.7698) (-5.4731, 3.7705) (-5.4881, 3.7712) (-5.505, 3.7718) (-5.5163, 3.7722) (-5.5276, 3.7726) (-5.5428, 3.773) (-5.5581, 3.7734) (-5.5715, 3.7736) (-5.585, 3.7738) (-5.5985, 3.774) (-5.6082, 3.7741) (-5.6179, 3.7741) (-5.6277, 3.7742) (-5.6375, 3.7742) (-5.6473, 3.7742) (-5.6571, 3.7742) (-5.667, 3.7741) (-5.6769, 3.774) (-5.6868, 3.7739) (-5.6967, 3.7738) (-5.7067, 3.7736) (-5.7167, 3.7734) (-5.7267, 3.7732) (-5.7368, 3.7729) (-5.7468, 3.7727) (-5.757, 3.7724) (-5.7671, 3.772) (-5.7772, 3.7717) (-5.7874, 3.7713) (-5.7976, 3.7709) (-5.8079, 3.7705) (-5.8181, 3.77) (-5.8284, 3.7695) (-5.8387, 3.769) (-5.849, 3.7685) (-5.8635, 3.7677) (-5.876, 3.7669) (-5.8864, 3.7663) (-5.8948, 3.7657) (-5.901, 3.7653) knots 0 0 0 0 0 0 0.004167 0.008333 0.0125 0.016667 0.020833 0.025 0.029167 0.033333 0.0375 0.041667 0.045833 0.05 0.054167 0.058333 0.0625 0.066667 0.070833 0.075 0.079167 0.083333 0.0875 0.091667 0.095833 0.1 0.104167 0.108333 0.1125 0.116667 0.120833 0.125 0.129167 0.1375 0.141667 0.145833 0.154167 0.158333 0.1625 0.170833 0.175 0.179167 0.183333 0.191667 0.208333 0.2125 0.216667 0.220833 0.229167 0.2375 0.241667 0.245833 0.254167 0.258333 0.2625 0.270833 0.275 0.279167 0.2875 0.291667 0.295833 0.304167 0.308333 0.3125 0.320833 0.325 0.329167 0.3375 0.341667 0.345833 0.354167 0.358333 0.3625 0.370833 0.375 0.379167 0.3875 0.391667 0.395833 0.404167 0.408333 0.4125 0.420833 0.425 0.429167 0.4375 0.441667 0.445833 0.454167 0.458333 0.4625 0.470833 0.475 0.479167 0.4875 0.491667 0.495833 0.504167 0.508333 0.5125 0.520833 0.525 0.529167 0.5375 0.541667 0.545833 0.554167 0.558333 0.5625 0.570833 0.575 0.579167 0.5875 0.591667 0.595833 0.604167 0.608333 0.6125 0.620833 0.625 0.629167 0.6375 0.641667 0.645833 0.654167 0.658333 0.6625 0.670833 0.675 0.679167 0.6875 0.691667 0.695833 0.704167 0.708333 0.7125 0.720833 0.725 0.729167 0.7375 0.741667 0.745833 0.754167 0.758333 0.7625 0.770833 0.775 0.779167 0.791667 0.795833 0.8 0.804167 0.808333 0.825 0.829167 0.833333 0.8375 0.845833 0.85 0.854167 0.866667 0.870833 0.875 0.879167 0.883333 0.8875 0.891667 0.895833 0.9 0.904167 0.908333 0.9125 0.916667 0.920833 0.925 0.929167 0.933333 0.9375 0.941667 0.945833 0.95 0.954167 0.958333 0.9625 0.966667 0.970833 0.975 0.979167 0.983333 0.9875 1 1 1 1 1 1
  arc A11 (-5.901, 3.7653) -> (-6.2114, 3.2278) centre (0, 0) ccw
  spline S12 degree 5 poles (-6.2114, 3.2278) (-6.2086, 3.2221) (-6.2049, 3.2146) (-6.2003, 3.2053) (-6.1947, 3.1941) (-6.1881, 3.1812) (-6.1834, 3.172) (-6.1787, 3.1628) (-6.174, 3.1536) (-6.1692, 3.1445) (-6.1645, 3.1354) (-6.1598, 3.1264) (-6.155, 3.1174) (-6.1502, 3.1084) (-6.1454, 3.0995) (-6.1406, 3.0906) (-6.1358, 3.0817) (-6.131, 3.0729) (-6.1262, 3.0641) (-6.1214, 3.0554) (-6.1165, 3.0466) (-6.1117, 3.038) (-6.1068, 3.0293) (-6.1019, 3.0207) (-6.0971, 3.0121) (-6.0922, 3.0036) (-6.0873, 2.9951) (-6.0824, 2.9866) (-6.0775, 2.9782) (-6.0726, 2.9698) (-6.0666, 2.9598) (-6.0607, 2.9498) (-6.0548, 2.9399) (-6.0478, 2.9284) (-6.0409, 2.917) (-6.0349, 2.9072) (-6.0289, 2.8975) (-6.023, 2.8879) (-6.017, 2.8783) (-6.011, 2.8688) (-6.0049, 2.8593) (-5.9979, 2.8484) (-5.9909, 2.8375) (-5.9849, 2.8282) (-5.9778, 2.8174) (-5.9707, 2.8067) (-5.9647, 2.7976) (-5.9576, 2.7871) (-5.9505, 2.7766) (-5.9445, 2.7677) (-5.9364, 2.7558) (-5.9283, 2.7441) (-5.9212, 2.734) (-5.914, 2.7239) (-5.9049, 2.711) (-5.8978, 2.7011) (-5.8907, 2.6912) (-5.8836, 2.6815) (-5.8744, 2.669) (-5.8673, 2.6594) (-5.8602, 2.6499) (-5.852, 2.6391) (-5.8439, 2.6285) (-5.8378, 2.6205) (-5.8307, 2.6113) (-5.8236, 2.6022) (-5.8175, 2.5945) (-5.8104, 2.5855) (-5.8033, 2.5766) (-5.7972, 2.569) (-5.7902, 2.5603) (-5.7831, 2.5516) (-5.777, 2.5442) (-5.77, 2.5357) (-5.7629, 2.5272) (-5.7569, 2.5201) (-5.7498, 2.5117) (-5.7428, 2.5035) (-5.7368, 2.4965) (-5.7298, 2.4885) (-5.7228, 2.4805) (-5.7168, 2.4737) (-5.7099, 2.4658) (-5.7029, 2.458) (-5.697, 2.4514) (-5.69, 2.4438) (-5.6831, 2.4362) (-5.6772, 2.4298) (-5.6704, 2.4224) (-5.6635, 2.4151) (-5.6577, 2.4089) (-5.6508, 2.4017) (-5.644, 2.3946) (-5.6382, 2.3886) (-5.6315, 2.3817) (-5.6248, 2.3748) (-5.619, 2.369) (-5.6123, 2.3623) (-5.6057, 2.3556) (-5.6, 2.35) (-5.5934, 2.3435) (-5.5868, 2.3371) (-5.5812, 2.3317) (-5.5746, 2.3254) (-5.5681, 2.3192) (-5.5626, 2.314) (-5.5561, 2.308) (-5.5497, 2.302) (-5.5443, 2.297) (-5.5379, 2.2912) (-5.5316, 2.2855) (-5.5262, 2.2806) (-5.52, 2.2751) (-5.5138, 2.2696) (-5.5085, 2.2649) (-5.5023, 2.2596) (-5.4962, 2.2543) (-5.491, 2.2499) (-5.485, 2.2448) (-5.4791, 2.2398) (-5.474, 2.2355) (-5.4681, 2.2306) (-5.4622, 2.2258) (-5.4572, 2.2218) (-5.4515, 2.2171) (-5.4458, 2.2126) (-5.4409, 2.2087) (-5.4353, 2.2043) (-5.4297, 2.1999) (-5.425, 2.1963) (-5.4195, 2.1921) (-5.4141, 2.188) (-5.4095, 2.1845) (-5.4042, 2.1806) (-5.399, 2.1767) (-5.3945, 2.1734) (-5.3894, 2.1697) (-5.3843, 2.166) (-5.38, 2.1629) (-5.375, 2.1594) (-5.3701, 2.156) (-5.366, 2.1531) (-5.3612, 2.1498) (-5.3565, 2.1466) (-5.3525, 2.1439) (-5.348, 2.1409) (-5.3435, 2.1379) (-5.3397, 2.1354) (-5.3353, 2.1326) (-5.331, 2.1298) (-5.3274, 2.1275) (-5.3232, 2.1249) (-5.3192, 2.1224) (-5.3158, 2.1202) (-5.3124, 2.1182) (-5.308, 2.1155) (-5.3043, 2.1133) (-5.3001, 2.1108) (-5.296, 2.1084) (-5.2921, 2.1062) (-5.2893, 2.1045) (-5.2865, 2.1029) (-5.2842, 2.1017) (-5.2819, 2.1004) (-5.2798, 2.0992) (-5.2776, 2.0981) (-5.2756, 2.0969) (-5.2735, 2.0958) (-5.2716, 2.0948) (-5.2696, 2.0938) (-5.2678, 2.0928) (-5.266, 2.0918) (-5.2642, 2.0909) (-5.2625, 2.0901) (-5.2609, 2.0892) (-5.2593, 2.0884) (-5.2577, 2.0877) (-5.2563, 2.087) (-5.2549, 2.0863) (-5.2535, 2.0856) (-5.2522, 2.085) (-5.251, 2.0844) (-5.2498, 2.0839) (-5.2487, 2.0834) (-5.2477, 2.0829) (-5.2467, 2.0824) (-5.2458, 2.082) (-5.245, 2.0817) (-5.2442, 2.0813) (-5.2435, 2.081) (-5.2429, 2.0807) (-5.2422, 2.0805) (-5.2418, 2.0803) (-5.2415, 2.0801) (-5.2413, 2.08) (-5.2411, 2.08) knots -1 -1 -1 -1 -1 -1 -0.9875 -0.983333 -0.979167 -0.975 -0.970833 -0.966667 -0.9625 -0.958333 -0.954167 -0.95 -0.945833 -0.941667 -0.9375 -0.933333 -0.929167 -0.925 -0.920833 -0.916667 -0.9125 -0.908333 -0.904167 -0.9 -0.895833 -0.891667 -0.8875 -0.883333 -0.879167 -0.875 -0.870833 -0.8625 -0.858333 -0.854167 -0.845833 -0.841667 -0.8375 -0.833333 -0.829167 -0.820833 -0.816667 -0.8125 -0.804167 -0.8 -0.795833 -0.7875 -0.783333 -0.779167 -0.770833 -0.766667 -0.7625 -0.75 -0.745833 -0.741667 -0.7375 -0.725 -0.720833 -0.716667 -0.7125 -0.7 -0.695833 -0.691667 -0.683333 -0.679167 -0.675 -0.666667 -0.6625 -0.658333 -0.65 -0.645833 -0.641667 -0.633333 -0.629167 -0.625 -0.616667 -0.6125 -0.608333 -0.6 -0.595833 -0.591667 -0.583333 -0.579167 -0.575 -0.566667 -0.5625 -0.558333 -0.55 -0.545833 -0.541667 -0.533333 -0.529167 -0.525 -0.516667 -0.5125 -0.508333 -0.5 -0.495833 -0.491667 -0.483333 -0.479167 -0.475 -0.466667 -0.4625 -0.458333 -0.45 -0.445833 -0.441667 -0.433333 -0.429167 -0.425 -0.416667 -0.4125 -0.408333 -0.4 -0.395833 -0.391667 -0.383333 -0.379167 -0.375 -0.366667 -0.3625 -0.358333 -0.35 -0.345833 -0.341667 -0.333333 -0.329167 -0.325 -0.316667 -0.3125 -0.308333 -0.3 -0.295833 -0.291667 -0.283333 -0.279167 -0.275 -0.266667 -0.2625 -0.258333 -0.25 -0.245833 -0.241667 -0.233333 -0.229167 -0.225 -0.216667 -0.2125 -0.208333 -0.2 -0.195833 -0.191667 -0.183333 -0.179167 -0.175 -0.170833 -0.158333 -0.154167 -0.145833 -0.141667 -0.1375 -0.133333 -0.129167 -0.125 -0.120833 -0.116667 -0.1125 -0.108333 -0.104167 -0.1 -0.095833 -0.091667 -0.0875 -0.083333 -0.079167 -0.075 -0.070833 -0.066667 -0.0625 -0.058333 -0.054167 -0.05 -0.045833 -0.041667 -0.0375 -0.033333 -0.029167 -0.025 -0.020833 -0.016667 -0.0125 -0.008333 0 0 0 0 0 0
  line L12 (-5.2411, 2.08) -> (-4.415, 1.7521)
  arc A12 (-4.415, 1.7521) -> (-4.6996, 0.6901) centre (0, 0) ccw
  line L13 (-4.6996, 0.6901) -> (-5.579, 0.8192)
  spline S13 degree 5 poles (-5.579, 0.8192) (-5.579, 0.8193) (-5.5792, 0.8193) (-5.5794, 0.8193) (-5.5797, 0.8193) (-5.5803, 0.8194) (-5.5809, 0.8195) (-5.5815, 0.8196) (-5.5823, 0.8196) (-5.5831, 0.8197) (-5.584, 0.8198) (-5.585, 0.8199) (-5.5861, 0.82) (-5.5872, 0.8201) (-5.5884, 0.8202) (-5.5897, 0.8203) (-5.5911, 0.8204) (-5.5925, 0.8206) (-5.594, 0.8207) (-5.5955, 0.8208) (-5.5972, 0.8209) (-5.5989, 0.821) (-5.6007, 0.8211) (-5.6025, 0.8212) (-5.6044, 0.8213) (-5.6064, 0.8214) (-5.6084, 0.8215) (-5.6105, 0.8216) (-5.6127, 0.8216) (-5.6149, 0.8217) (-5.6172, 0.8218) (-5.6196, 0.8218) (-5.6225, 0.8219) (-5.6255, 0.822) (-5.6286, 0.822) (-5.6323, 0.822) (-5.6362, 0.8221) (-5.6396, 0.8221) (-5.6437, 0.8221) (-5.6478, 0.822) (-5.6515, 0.822) (-5.6559, 0.8219) (-5.6604, 0.8218) (-5.6644, 0.8217) (-5.6691, 0.8215) (-5.6739, 0.8214) (-5.6781, 0.8212) (-5.6831, 0.821) (-5.6883, 0.8207) (-5.6927, 0.8205) (-5.6981, 0.8202) (-5.7035, 0.8198) (-5.7082, 0.8195) (-5.7138, 0.8191) (-5.7195, 0.8187) (-5.7245, 0.8183) (-5.7304, 0.8178) (-5.7364, 0.8172) (-5.7416, 0.8168) (-5.7477, 0.8162) (-5.754, 0.8155) (-5.7594, 0.8149) (-5.7658, 0.8142) (-5.7723, 0.8135) (-5.778, 0.8128) (-5.7847, 0.812) (-5.7915, 0.8111) (-5.7973, 0.8103) (-5.8042, 0.8094) (-5.8113, 0.8084) (-5.8173, 0.8075) (-5.8245, 0.8064) (-5.8318, 0.8053) (-5.8381, 0.8043) (-5.8455, 0.8031) (-5.853, 0.8019) (-5.8594, 0.8008) (-5.8671, 0.7995) (-5.8748, 0.7981) (-5.8814, 0.7969) (-5.8893, 0.7954) (-5.8972, 0.7939) (-5.9041, 0.7925) (-5.9122, 0.7909) (-5.9203, 0.7892) (-5.9273, 0.7878) (-5.9356, 0.786) (-5.944, 0.7842) (-5.9512, 0.7826) (-5.9596, 0.7807) (-5.9682, 0.7787) (-5.9756, 0.777) (-5.9842, 0.775) (-5.993, 0.7728) (-6.0005, 0.771) (-6.0094, 0.7688) (-6.0183, 0.7665) (-6.026, 0.7645) (-6.035, 0.7621) (-6.0441, 0.7597) (-6.052, 0.7576) (-6.0612, 0.755) (-6.0705, 0.7524) (-6.0785, 0.7501) (-6.0879, 0.7474) (-6.0973, 0.7447) (-6.1055, 0.7423) (-6.115, 0.7394) (-6.1246, 0.7365) (-6.1329, 0.7339) (-6.1426, 0.7309) (-6.1524, 0.7277) (-6.1608, 0.725) (-6.1707, 0.7218) (-6.1806, 0.7185) (-6.1892, 0.7157) (-6.1992, 0.7123) (-6.2093, 0.7088) (-6.2179, 0.7058) (-6.2281, 0.7023) (-6.2383, 0.6986) (-6.2471, 0.6955) (-6.2574, 0.6917) (-6.2677, 0.6879) (-6.2766, 0.6846) (-6.2871, 0.6807) (-6.2976, 0.6767) (-6.3066, 0.6732) (-6.3171, 0.6691) (-6.3277, 0.6649) (-6.3369, 0.6613) (-6.3475, 0.657) (-6.3583, 0.6526) (-6.3675, 0.6488) (-6.3783, 0.6443) (-6.3891, 0.6398) (-6.3985, 0.6358) (-6.4094, 0.6312) (-6.4203, 0.6264) (-6.4298, 0.6223) (-6.4408, 0.6175) (-6.4518, 0.6125) (-6.4614, 0.6082) (-6.4725, 0.6032) (-6.4837, 0.5981) (-6.4933, 0.5936) (-6.5045, 0.5884) (-6.5157, 0.5831) (-6.5254, 0.5785) (-6.5351, 0.5738) (-6.5497, 0.5667) (-6.5627, 0.5604) (-6.5758, 0.5539) (-6.5889, 0.5473) (-6.6053, 0.539) (-6.6169, 0.5331) (-6.6285, 0.5271) (-6.64, 0.521) (-6.655, 0.5131) (-6.6666, 0.5069) (-6.6783, 0.5006) (-6.6917, 0.4934) (-6.7051, 0.486) (-6.7152, 0.4804) (-6.7253, 0.4748) (-6.7354, 0.4691) (-6.7439, 0.4644) (-6.7523, 0.4595) (-6.7608, 0.4547) (-6.7693, 0.4498) (-6.7778, 0.4449) (-6.7863, 0.44) (-6.7948, 0.435) (-6.8033, 0.43) (-6.8118, 0.4249) (-6.8204, 0.4198) (-6.8289, 0.4147) (-6.8375, 0.4095) (-6.8461, 0.4043) (-6.8547, 0.3991) (-6.8632, 0.3938) (-6.8718, 0.3885) (-6.8805, 0.3831) (-6.8891, 0.3778) (-6.8977, 0.3723) (-6.9063, 0.3669) (-6.915, 0.3614) (-6.9236, 0.3559) (-6.9323, 0.3503) (-6.941, 0.3447) (-6.9496, 0.3391) (-6.9618, 0.3311) (-6.9722, 0.3243) (-6.9809, 0.3185) (-6.9879, 0.3138) (-6.9931, 0.3103) knots 0 0 0 0 0 0 0.004167 0.008333 0.0125 0.016667 0.020833 0.025 0.029167 0.033333 0.0375 0.041667 0.045833 0.05 0.054167 0.058333 0.0625 0.066667 0.070833 0.075 0.079167 0.083333 0.0875 0.091667 0.095833 0.1 0.104167 0.108333 0.1125 0.116667 0.120833 0.125 0.129167 0.1375 0.141667 0.145833 0.154167 0.158333 0.1625 0.170833 0.175 0.179167 0.1875 0.191667 0.195833 0.204167 0.208333 0.2125 0.220833 0.225 0.229167 0.2375 0.241667 0.245833 0.254167 0.258333 0.2625 0.270833 0.275 0.279167 0.2875 0.291667 0.295833 0.304167 0.308333 0.3125 0.320833 0.325 0.329167 0.3375 0.341667 0.345833 0.354167 0.358333 0.3625 0.370833 0.375 0.379167 0.3875 0.391667 0.395833 0.404167 0.408333 0.4125 0.420833 0.425 0.429167 0.4375 0.441667 0.445833 0.454167 0.458333 0.4625 0.470833 0.475 0.479167 0.4875 0.491667 0.495833 0.504167 0.508333 0.5125 0.520833 0.525 0.529167 0.5375 0.541667 0.545833 0.554167 0.558333 0.5625 0.570833 0.575 0.579167 0.5875 0.591667 0.595833 0.604167 0.608333 0.6125 0.620833 0.625 0.629167 0.6375 0.641667 0.645833 0.654167 0.658333 0.6625 0.670833 0.675 0.679167 0.6875 0.691667 0.695833 0.704167 0.708333 0.7125 0.720833 0.725 0.729167 0.7375 0.741667 0.745833 0.754167 0.758333 0.7625 0.770833 0.775 0.779167 0.783333 0.8 0.804167 0.808333 0.8125 0.825 0.829167 0.833333 0.8375 0.85 0.854167 0.858333 0.866667 0.870833 0.875 0.879167 0.883333 0.8875 0.891667 0.895833 0.9 0.904167 0.908333 0.9125 0.916667 0.920833 0.925 0.929167 0.933333 0.9375 0.941667 0.945833 0.95 0.954167 0.958333 0.9625 0.966667 0.970833 0.975 0.979167 0.983333 0.9875 1 1 1 1 1 1
  arc A13 (-6.9931, 0.3103) -> (-6.9931, -0.3103) centre (0, 0) ccw